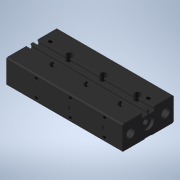
# Autodesk Inventor part: 170831 DFM-12-100-P-A-GF---(Z)
Saved by Autodesk Inventor 2021 (Build 250183000, 183)
## iProperties
Created: 2025-06-15
Part Number: 170831 DFM-12-100-P-A-GF---(Z)
Material: Generic
Catalog Web Link: www.cadenas.de
Description: DFM-(Z)-Guide unit
Vendor: FESTO
Document SubType Name: Modeling
Designer: psAdmin
Manufacturer: FESTO
Mass: 180.298 g
Surface Area: 463.67 cm^2
Volume: 180.298 cm^3
Density: 1 g/cm^3
Appearance: PSOLRGB-175-175-175
Category: PARTsolutions
Company: FESTO
Title: 170831 DFM-12-100-P-A-GF---(Z)
Author: Cadenas PARTsolutions
Comments: Guide unit
PSOL_IDENT_0: {$CADENAS_DATA/23d-libs/festo_fdt/parts/d/dfm/parts/dfm_z.prj},201 {VTYP=3D},{NB=170831 DFM-12-100-P
PSOL_IDENT_1: -A-GF---(Z)},{LINA=170831 DFM-12-100-P-A-GF---(Z)},{NN=DFM-(Z)},{DATE=04.04.2025 09:42:25},{GEOMDATE=
PSOL_IDENT_2: 20.01.2025 12:21:39},{VERSION=},{LINEID=80},{WBVAR=},{WBNUMERIC=}  {NB=170831 DFM-12-100-P-A-GF---(Z
PSOL_IDENT_3: )},{LINA=170831 DFM-12-100-P-A-GF---(Z)},{KT=1},{TNR=170831},{TYP=DFM},{KDM=12},{HUB=100},{F=GF},{BW
PSOL_IDENT_4: E=-},{B1=60.000},{B2=58.000},{B3=42.400},{B4=30.000},{B5=4.500},{B6=51.000},{B7=20.500},{B8=19.000},
PSOL_IDENT_5: {B9=20.000},{B10=20.000},{B11=9.500},{B12=41.000},{B13=19.500},{B14=21.000},{D1=M 5},{D1P=5.000},{D1
PSOL_IDENT_6: KDR=4.134},{D2=8.000},{D3=9.000},{D4=M 4},{D4P=4.000},{D4KDR=3.242},{D5=0.000},{D6=M 4},{D6P=4.000},
PSOL_IDENT_7: {D6KDR=3.242},{D7=10},{D7GF=10.000},{D7KF=8.000},{D8=5.000},{D9=4.300},{FN=1},{FT=GF},{BWET=},{EE=M
PSOL_IDENT_8: 5},{EEMM=5.000},{EEKDR=4.134},{H1=28.050},{H2=26.000},{H3=24.000},{H4=14.050},{H5=14.050},{H6=4.000}
PSOL_IDENT_9: ,{H7=20.000},{H8=0.000},{H9=4.000},{H10=20.000},{H11=14.000},{L1=155.000},{L2=136.000},{L3=10.000},{
PSOL_IDENT_10: L4=13.000},{L5=11.400},{L6=9.500},{L7=6.000},{L8=21.000},{L9=40.000},{L10=34.000},{L11=80.000},{L12=
PSOL_IDENT_11: 11.400},{T1=9.000},{T2=9.400},{T3=2.100},{T4=8.000},{T5=0.000},{T6=1.000},{SW1=14.000},{SW2=11.000},
PSOL_IDENT_12: {SW2D=6.000},{SW2T=3.200},{ZZ=0},{MOD=1},{NA=8.000},{BM=0.000},{BS=0.000},{FE=1.000},{A1=5.000},{A2=
PSOL_IDENT_13: 8.600},{W=30.000},{BR=8.000},{D10=14},{A3=3}
NB: 170831 DFM-12-100-P-A-GF---(Z)
NN: DFM-(Z)
NT: Guide unit
NBSYN: $TNR. $TYP.-$KDM.-$HUB.-P-A-$FT.$BWET.---(Z)
LINA: 170831 DFM-12-100-P-A-GF---(Z)
CATALOG: Festo Design Tool 3D
TNR: 170831
TYP: DFM
KDM: 12
HUB: 100
F: GF
BWE: -
B1: 60
B2: 58
B3: 42.4
B4: 30
B5: 4.5
B6: 51
B7: 20.5
B8: 19
B9: 20
B10: 20
B11: 9.5
B12: 41
B13: 19.5
B14: 21
D1: M 5
D1P: 5
D1KDR: 4.134
D2: 8
D3: 9
D4: M 4
D4P: 4
D4KDR: 3.242
D5: 0
D6: M 4
D6P: 4
D6KDR: 3.242
D7GF: 10
D7KF: 8
D8: 5
D9: 4.3
EE: M 5
EEKDR: 4.134
H1: 28.05
H2: 26
H3: 24
H4: 14.05
H5: 14.05
H6: 4
H7: 20
H8: 0
H9: 4
H10: 20
H11: 14
L1: 155
L2: 136
L3: 10
L4: 13
L5: 11.4
L6: 9.5
L7: 6
L8: 21
L9: 40
L10: 34
L11: 80
L12: 11.4
T1: 9
T2: 9.4
T3: 2.1
T4: 8
T5: 0
T6: 1
SW1: 14
SW2: 11
SW2D: 6
SW2T: 3.2
NA: 8
BM: 0
BS: 0
FE: 1
A1: 5
A2: 8.6
W: 30
BR: 8
SUPPLIER: FESTO
ARTICLENO: 170831 DFM-12-100-P-A-GF---(Z)
BOMINFO: 170831 DFM-12-100-P-A-GF---(Z)
CREATOR: CADENAS GmbH
Autodesk Inventor part; units mm, degrees
ref_plane "YZ Plane" through (0, 0, 0) normal (1, 0, 0) x (0, 1, 0)
ref_plane "XZ Plane" through (0, 0, 0) normal (0, 1, 0) x (-1, 0, 0)
ref_plane "XY Plane" through (0, 0, 0) normal (0, 0, 1) x (1, 0, 0)
sketch "Sketch_1" plane through (0, 0, 0) normal (1, 0, 0) x (0, 1, 0)
  line L0 (14, 30) -> (-14.05, 30)
  line L1 (-14.05, 30) -> (-14.05, -30)
  line L2 (-14.05, -30) -> (14, -30)
  line L3 (14, -30) -> (14, 30)
  constraints: 8 end point
extrude "Extrusion1" add sketch "Sketch_1" against normal blind 136
sketch "Sketch_37" plane through (0, 0, 0) normal (1, 0, 0) x (0, 1, 0)
  line L0 (-40, 60) -> (-40, -60)
  line L1 (-40, -60) -> (40, -60)
  line L2 (40, -60) -> (40, 60)
  line L3 (40, 60) -> (-40, 60)
  line L4 (-13.5, 30) -> (-14.05, 29.45)
  line L5 (-14.05, 29.45) -> (-14.05, 4.0402)
  line L6 (-14.05, 4.0402) -> (-13.5, 3.7226)
  line L7 (-13.5, 3.7226) -> (-13.5, -3.7226)
  line L8 (-13.5, -3.7226) -> (-14.05, -4.0402)
  line L9 (-14.05, -4.0402) -> (-14.05, -28.95)
  line L10 (-14.05, -28.95) -> (-13, -30)
  line L11 (-13, -30) -> (13, -30)
  line L12 (13, -30) -> (14, -29)
  line L13 (14, -29) -> (14, -7)
  arc A0 (14, -7) -> (13.6, -6.6) centre (13.6, -7) ccw
  line L14 (13.6, -6.6) -> (12.4, -6.6)
  arc A1 (12.4, -6.6) -> (12.2, -6.8) centre (12.4, -6.8) ccw
  line L15 (12.2, -6.8) -> (12.2, -7.05)
  arc A2 (12, -7.25) -> (12.2, -7.05) centre (12, -7.05) ccw
  line L16 (12, -7.25) -> (9.4, -7.25)
  arc A3 (9, -6.85) -> (9.4, -7.25) centre (9.4, -6.85) ccw
  line L17 (9, -6.85) -> (9, -1.15)
  arc A4 (9.4, -0.75) -> (9, -1.15) centre (9.4, -1.15) ccw
  line L18 (9.4, -0.75) -> (12, -0.75)
  arc A5 (12.2, -0.95) -> (12, -0.75) centre (12, -0.95) ccw
  line L19 (12.2, -0.95) -> (12.2, -1.2)
  arc A6 (12.2, -1.2) -> (12.4, -1.4) centre (12.4, -1.2) ccw
  line L20 (12.4, -1.4) -> (13.6, -1.4)
  arc A7 (13.6, -1.4) -> (14, -1) centre (13.6, -1) ccw
  line L21 (14, -1) -> (14, 1)
  arc A8 (14, 1) -> (13.6, 1.4) centre (13.6, 1) ccw
  line L22 (13.6, 1.4) -> (12.4, 1.4)
  arc A9 (12.4, 1.4) -> (12.2, 1.2) centre (12.4, 1.2) ccw
  line L23 (12.2, 1.2) -> (12.2, 0.95)
  arc A10 (12, 0.75) -> (12.2, 0.95) centre (12, 0.95) ccw
  line L24 (12, 0.75) -> (9.4, 0.75)
  arc A11 (9, 1.15) -> (9.4, 0.75) centre (9.4, 1.15) ccw
  line L25 (9, 1.15) -> (9, 6.85)
  arc A12 (9.4, 7.25) -> (9, 6.85) centre (9.4, 6.85) ccw
  line L26 (9.4, 7.25) -> (12, 7.25)
  arc A13 (12.2, 7.05) -> (12, 7.25) centre (12, 7.05) ccw
  line L27 (12.2, 7.05) -> (12.2, 6.8)
  arc A14 (12.2, 6.8) -> (12.4, 6.6) centre (12.4, 6.8) ccw
  line L28 (12.4, 6.6) -> (13.6, 6.6)
  arc A15 (13.6, 6.6) -> (14, 7) centre (13.6, 7) ccw
  line L29 (14, 7) -> (14, 29)
  line L30 (14, 29) -> (13, 30)
  line L31 (13, 30) -> (-13.5, 30)
  constraints: 64 end point, 32 point on circle, 16 centre point
extrude "Extrusion2" cut sketch "Sketch_37" against normal blind 136
sketch "Sketch3" plane through (0, 0, 0) normal (1, 0, 0) x (0, 0, -1)
  point P0 (20.5, 0)
hole "Hole1" at (0, 0, -20.5) direction (-1, 0, 0) diameter 10 depth 136
sketch "Sketch4" plane through (0, 0, 0) normal (1, 0, 0) x (0, 0, -1)
  point P0 (-20.5, 0)
hole "Hole2" at (0, 0, 20.5) direction (-1, 0, 0) diameter 10 depth 136
sketch "Sketch5" plane through (-136, 14, -29) normal (0, 1, 0) x (1, 0, 0)
  point P0 (124.6, -16.6)
hole "Hole3" at (-11.4, 14, -12.4) direction (0, -1, 0) diameter 4.134 depth 5 countersink diameter 5 countersink angle 90 thread size "M5x0.8" class "6H" standard "ISO Metric profile"
sketch "Sketch6" plane through (-136, 14, -29) normal (0, 1, 0) x (1, 0, 0)
  point P0 (9.5, -16.6)
hole "Hole4" at (-126.5, 14, -12.4) direction (0, -1, 0) diameter 4.134 depth 5 countersink diameter 5 countersink angle 90 thread size "M5x0.8" class "6H" standard "ISO Metric profile"
sketch "Sketch7" plane through (0, -13, -30) normal (0, 0, -1) x (-1, 0, 0)
  point P0 (11.4, 22.95)
hole "Hole5" at (-11.4, 9.95, -30) direction (0, 0, 1) diameter 4.134 depth 5 countersink diameter 5 countersink angle 90 thread size "M5x0.8" class "6H" standard "ISO Metric profile"
sketch "Sketch8" plane through (0, -13, -30) normal (0, 0, -1) x (-1, 0, 0)
  point P0 (126.5, 22.95)
hole "Hole6" at (-126.5, 9.95, -30) direction (0, 0, 1) diameter 4.134 depth 5 countersink diameter 5 countersink angle 90 thread size "M5x0.8" class "6H" standard "ISO Metric profile"
sketch "Sketch_18" plane through (-21, 0, 0) normal (1, 0, 0) x (0, 0, -1)
  line L0 (9.5, -14.05) -> (9.5, 14)
  line L1 (9.5, 14) -> (13.5, 14)
  line L2 (13.5, 14) -> (13.5, 4.6)
  line L3 (13.5, 4.6) -> (11.65, 4.6)
  line L4 (11.65, 4.6) -> (11.65, -5.05)
  line L5 (11.65, -5.05) -> (10.5, -5.05)
  line L6 (10.5, -5.05) -> (10.5, -11.95)
  line L7 (10.5, -11.95) -> (14, -11.95)
  line L8 (14, -11.95) -> (14, -14.05)
  line L9 (14, -14.05) -> (9.5, -14.05)
  line L10 (9.5, -14.05) -> (9.5, 14)
  constraints: 22 end point
revolve "Revolution1" cut sketch "Sketch_18" angle 360 about axis through (-21, -14.05, -9.5) along (0, 1, 0)
sketch "Sketch_5" plane through (-21, 0, 0) normal (1, 0, 0) x (0, 0, -1)
  line L0 (9.5, -11.95) -> (9.5, -5.05)
  line L1 (9.5, -5.05) -> (11.567, -5.05)
  line L2 (11.567, -5.05) -> (11.567, -11.517)
  line L3 (11.567, -11.517) -> (12, -11.95)
  line L4 (12, -11.95) -> (9.5, -11.95)
  line L5 (9.5, -11.95) -> (9.5, -5.05)
  constraints: 12 end point
revolve "Revolution2" cut sketch "Sketch_5" angle 360 about axis through (-21, -11.95, -9.5) along (0, 1, 0)
thread "Thread1" size "M5x0.8" class "6H" standard "ISO Metric profile" full length
sketch "Sketch_19" plane through (-21, 0, 0) normal (1, 0, 0) x (0, 0, -1)
  line L0 (-9.5, -14.05) -> (-9.5, 14)
  line L1 (-9.5, 14) -> (-5.5, 14)
  line L2 (-5.5, 14) -> (-5.5, 4.6)
  line L3 (-5.5, 4.6) -> (-7.35, 4.6)
  line L4 (-7.35, 4.6) -> (-7.35, -5.05)
  line L5 (-7.35, -5.05) -> (-8.5, -5.05)
  line L6 (-8.5, -5.05) -> (-8.5, -11.95)
  line L7 (-8.5, -11.95) -> (-5, -11.95)
  line L8 (-5, -11.95) -> (-5, -14.05)
  line L9 (-5, -14.05) -> (-9.5, -14.05)
  line L10 (-9.5, -14.05) -> (-9.5, 14)
  constraints: 22 end point
revolve "Revolution3" cut sketch "Sketch_19" angle 360 about axis through (-21, -14.05, 9.5) along (0, 1, 0)
sketch "Sketch_6" plane through (-21, 0, 0) normal (1, 0, 0) x (0, 0, -1)
  line L0 (-9.5, -11.95) -> (-9.5, -5.05)
  line L1 (-9.5, -5.05) -> (-7.433, -5.05)
  line L2 (-7.433, -5.05) -> (-7.433, -11.517)
  line L3 (-7.433, -11.517) -> (-7, -11.95)
  line L4 (-7, -11.95) -> (-9.5, -11.95)
  line L5 (-9.5, -11.95) -> (-9.5, -5.05)
  constraints: 12 end point
revolve "Revolution4" cut sketch "Sketch_6" angle 360 about axis through (-21, -11.95, 9.5) along (0, 1, 0)
thread "Thread2" size "M5x0.8" class "6H" standard "ISO Metric profile" full length
sketch "Sketch_20" plane through (-61, 0, 0) normal (1, 0, 0) x (0, 0, -1)
  line L0 (9.5, -14.05) -> (9.5, 14)
  line L1 (9.5, 14) -> (13.5, 14)
  line L2 (13.5, 14) -> (13.5, 4.6)
  line L3 (13.5, 4.6) -> (11.65, 4.6)
  line L4 (11.65, 4.6) -> (11.65, -5.05)
  line L5 (11.65, -5.05) -> (10.5, -5.05)
  line L6 (10.5, -5.05) -> (10.5, -14.05)
  line L7 (10.5, -14.05) -> (9.5, -14.05)
  line L8 (9.5, -14.05) -> (9.5, 14)
  constraints: 18 end point
revolve "Revolution5" cut sketch "Sketch_20" angle 360 about axis through (-61, -14.05, -9.5) along (0, 1, 0)
sketch "Sketch_7" plane through (-61, 0, 0) normal (1, 0, 0) x (0, 0, -1)
  line L0 (9.5, -14.05) -> (9.5, -5.05)
  line L1 (9.5, -5.05) -> (11.567, -5.05)
  line L2 (11.567, -5.05) -> (11.567, -13.617)
  line L3 (11.567, -13.617) -> (12, -14.05)
  line L4 (12, -14.05) -> (9.5, -14.05)
  line L5 (9.5, -14.05) -> (9.5, -5.05)
  constraints: 12 end point
revolve "Revolution6" cut sketch "Sketch_7" angle 360 about axis through (-61, -14.05, -9.5) along (0, 1, 0)
thread "Thread3" size "M5x0.8" class "6H" standard "ISO Metric profile" full length
sketch "Sketch_21" plane through (-61, 0, 0) normal (1, 0, 0) x (0, 0, -1)
  line L0 (-9.5, -14.05) -> (-9.5, 14)
  line L1 (-9.5, 14) -> (-5.5, 14)
  line L2 (-5.5, 14) -> (-5.5, 4.6)
  line L3 (-5.5, 4.6) -> (-7.35, 4.6)
  line L4 (-7.35, 4.6) -> (-7.35, -5.05)
  line L5 (-7.35, -5.05) -> (-8.5, -5.05)
  line L6 (-8.5, -5.05) -> (-8.5, -14.05)
  line L7 (-8.5, -14.05) -> (-9.5, -14.05)
  line L8 (-9.5, -14.05) -> (-9.5, 14)
  constraints: 18 end point
revolve "Revolution7" cut sketch "Sketch_21" angle 360 about axis through (-61, -14.05, 9.5) along (0, 1, 0)
sketch "Sketch_8" plane through (-61, 0, 0) normal (1, 0, 0) x (0, 0, -1)
  line L0 (-9.5, -14.05) -> (-9.5, -5.05)
  line L1 (-9.5, -5.05) -> (-7.433, -5.05)
  line L2 (-7.433, -5.05) -> (-7.433, -13.617)
  line L3 (-7.433, -13.617) -> (-7, -14.05)
  line L4 (-7, -14.05) -> (-9.5, -14.05)
  line L5 (-9.5, -14.05) -> (-9.5, -5.05)
  constraints: 12 end point
revolve "Revolution8" cut sketch "Sketch_8" angle 360 about axis through (-61, -14.05, 9.5) along (0, 1, 0)
thread "Thread4" size "M5x0.8" class "6H" standard "ISO Metric profile" full length
sketch "Sketch_22" plane through (-101, 0, 0) normal (1, 0, 0) x (0, 0, -1)
  line L0 (9.5, -14.05) -> (9.5, 14)
  line L1 (9.5, 14) -> (13.5, 14)
  line L2 (13.5, 14) -> (13.5, 4.6)
  line L3 (13.5, 4.6) -> (11.65, 4.6)
  line L4 (11.65, 4.6) -> (11.65, -5.05)
  line L5 (11.65, -5.05) -> (10.5, -5.05)
  line L6 (10.5, -5.05) -> (10.5, -14.05)
  line L7 (10.5, -14.05) -> (9.5, -14.05)
  line L8 (9.5, -14.05) -> (9.5, 14)
  constraints: 18 end point
revolve "Revolution9" cut sketch "Sketch_22" angle 360 about axis through (-101, -14.05, -9.5) along (0, 1, 0)
sketch "Sketch_9" plane through (-101, 0, 0) normal (1, 0, 0) x (0, 0, -1)
  line L0 (9.5, -14.05) -> (9.5, -5.05)
  line L1 (9.5, -5.05) -> (11.567, -5.05)
  line L2 (11.567, -5.05) -> (11.567, -13.617)
  line L3 (11.567, -13.617) -> (12, -14.05)
  line L4 (12, -14.05) -> (9.5, -14.05)
  line L5 (9.5, -14.05) -> (9.5, -5.05)
  constraints: 12 end point
revolve "Revolution10" cut sketch "Sketch_9" angle 360 about axis through (-101, -14.05, -9.5) along (0, 1, 0)
thread "Thread5" size "M5x0.8" class "6H" standard "ISO Metric profile" full length
sketch "Sketch_23" plane through (-101, 0, 0) normal (1, 0, 0) x (0, 0, -1)
  line L0 (-9.5, -14.05) -> (-9.5, 14)
  line L1 (-9.5, 14) -> (-5.5, 14)
  line L2 (-5.5, 14) -> (-5.5, 4.6)
  line L3 (-5.5, 4.6) -> (-7.35, 4.6)
  line L4 (-7.35, 4.6) -> (-7.35, -5.05)
  line L5 (-7.35, -5.05) -> (-8.5, -5.05)
  line L6 (-8.5, -5.05) -> (-8.5, -14.05)
  line L7 (-8.5, -14.05) -> (-9.5, -14.05)
  line L8 (-9.5, -14.05) -> (-9.5, 14)
  constraints: 18 end point
revolve "Revolution11" cut sketch "Sketch_23" angle 360 about axis through (-101, -14.05, 9.5) along (0, 1, 0)
sketch "Sketch_10" plane through (-101, 0, 0) normal (1, 0, 0) x (0, 0, -1)
  line L0 (-9.5, -14.05) -> (-9.5, -5.05)
  line L1 (-9.5, -5.05) -> (-7.433, -5.05)
  line L2 (-7.433, -5.05) -> (-7.433, -13.617)
  line L3 (-7.433, -13.617) -> (-7, -14.05)
  line L4 (-7, -14.05) -> (-9.5, -14.05)
  line L5 (-9.5, -14.05) -> (-9.5, -5.05)
  constraints: 12 end point
revolve "Revolution12" cut sketch "Sketch_10" angle 360 about axis through (-101, -14.05, 9.5) along (0, 1, 0)
thread "Thread6" size "M5x0.8" class "6H" standard "ISO Metric profile" full length
sketch "Sketch21" plane through (-136, -13.5, 30) normal (0, 0, 1) x (1, 0, 0)
  point P0 (115, 3.45)
hole "Hole7" at (-21, -10.05, 30) direction (0, 0, -1) diameter 3.242 depth 9.7308 tip angle 120 countersink diameter 4 countersink angle 90 thread size "M4x0.7" class "6H" standard "ISO Metric profile"
sketch "Sketch22" plane through (-136, -13.5, 30) normal (0, 0, 1) x (1, 0, 0)
  point P0 (115, 23.45)
hole "Hole8" at (-21, 9.95, 30) direction (0, 0, -1) diameter 3.242 depth 9.7308 tip angle 120 countersink diameter 4 countersink angle 90 thread size "M4x0.7" class "6H" standard "ISO Metric profile"
sketch "Sketch23" plane through (-136, -13.5, 30) normal (0, 0, 1) x (1, 0, 0)
  point P0 (75, 3.45)
hole "Hole9" at (-61, -10.05, 30) direction (0, 0, -1) diameter 3.242 depth 9.7308 tip angle 120 countersink diameter 4 countersink angle 90 thread size "M4x0.7" class "6H" standard "ISO Metric profile"
sketch "Sketch24" plane through (-136, -13.5, 30) normal (0, 0, 1) x (1, 0, 0)
  point P0 (75, 23.45)
hole "Hole10" at (-61, 9.95, 30) direction (0, 0, -1) diameter 3.242 depth 9.7308 tip angle 120 countersink diameter 4 countersink angle 90 thread size "M4x0.7" class "6H" standard "ISO Metric profile"
sketch "Sketch25" plane through (-136, -13.5, 30) normal (0, 0, 1) x (1, 0, 0)
  point P0 (35, 3.45)
hole "Hole11" at (-101, -10.05, 30) direction (0, 0, -1) diameter 3.242 depth 9.7308 tip angle 120 countersink diameter 4 countersink angle 90 thread size "M4x0.7" class "6H" standard "ISO Metric profile"
sketch "Sketch26" plane through (-136, -13.5, 30) normal (0, 0, 1) x (1, 0, 0)
  point P0 (35, 23.45)
hole "Hole12" at (-101, 9.95, 30) direction (0, 0, -1) diameter 3.242 depth 9.7308 tip angle 120 countersink diameter 4 countersink angle 90 thread size "M4x0.7" class "6H" standard "ISO Metric profile"
sketch "Sketch27" plane through (-136, 0, 0) normal (-1, 0, 0) x (0, 0, 1)
  point P0 (25.5, -10.05)
hole "Hole13" at (-136, -10.05, 25.5) direction (1, 0, 0) diameter 3.242 depth 9.7308 tip angle 120 countersink diameter 4 countersink angle 90 thread size "M4x0.7" class "6H" standard "ISO Metric profile"
sketch "Sketch28" plane through (-136, 0, 0) normal (-1, 0, 0) x (0, 0, 1)
  point P0 (25.5, 9.95)
hole "Hole14" at (-136, 9.95, 25.5) direction (1, 0, 0) diameter 3.242 depth 9.7308 tip angle 120 countersink diameter 4 countersink angle 90 thread size "M4x0.7" class "6H" standard "ISO Metric profile"
sketch "Sketch29" plane through (-136, 0, 0) normal (-1, 0, 0) x (0, 0, 1)
  point P0 (-25.5, -10.05)
hole "Hole15" at (-136, -10.05, -25.5) direction (1, 0, 0) diameter 3.242 depth 9.7308 tip angle 120 countersink diameter 4 countersink angle 90 thread size "M4x0.7" class "6H" standard "ISO Metric profile"
sketch "Sketch30" plane through (-136, 0, 0) normal (-1, 0, 0) x (0, 0, 1)
  point P0 (10.5, -0.05)
hole "Hole16" at (-136, -0.05, 10.5) direction (1, 0, 0) diameter 5 depth 1
sketch "Sketch31" plane through (-136, 0, 0) normal (-1, 0, 0) x (0, 0, 1)
  point P0 (-10.5, -0.05)
hole "Hole17" at (-136, -0.05, -10.5) direction (1, 0, 0) diameter 5 depth 1
sketch "Skizze_1" plane through (0, 0, 0) normal (0, 0, 1) x (1, 0, 0)
  line L0 (0, 0) -> (-117.4, 0)
  line L1 (-117.4, 0) -> (-117.4, 6)
  line L2 (-117.4, 6) -> (-11.4, 6)
  line L3 (-11.4, 6) -> (-11.4, 3)
  line L4 (-11.4, 3) -> (-3, 3)
  line L5 (-3, 3) -> (-3, 7)
  line L6 (-3, 7) -> (0, 7)
  line L7 (0, 7) -> (0, 0)
  line L8 (0, 0) -> (-117.4, 0)
  constraints: 18 end point
revolve "Revolution13" cut sketch "Skizze_1" angle 360 about axis through (0, 0, 0) along (1, 0, 0)
sketch "Skizze_5" plane through (-21, 0, 0) normal (1, 0, 0) x (0, 0, -1)
  line L0 (-29, -0.05) -> (-30, -0.05)
  line L1 (-30, -0.05) -> (-30, 2.45)
  line L2 (-30, 2.45) -> (-29, 2.45)
  line L3 (-29, 2.45) -> (-29, -0.05)
  line L4 (-29, -0.05) -> (-30, -0.05)
  constraints: 10 end point
revolve "Revolution14" cut sketch "Skizze_5" angle 360 about axis through (-21, -0.05, 29) along (0, 0, -1)
sketch "Skizze_6" plane through (-61, 0, 0) normal (1, 0, 0) x (0, 0, -1)
  line L0 (-29, -0.05) -> (-30, -0.05)
  line L1 (-30, -0.05) -> (-30, 2.45)
  line L2 (-30, 2.45) -> (-29, 2.45)
  line L3 (-29, 2.45) -> (-29, -0.05)
  line L4 (-29, -0.05) -> (-30, -0.05)
  constraints: 10 end point
revolve "Revolution15" cut sketch "Skizze_6" angle 360 about axis through (-61, -0.05, 29) along (0, 0, -1)
ref_plane "BP_1_XY" through (-11.4, 14, -12.4) normal (0, 1, 0) x (1, 0, 0)
ref_plane "BP_1_YZ" through (-11.4, 14, -12.4) normal (1, 0, 0) x (0, 0, -1)
ref_plane "BP_1_ZX" through (-11.4, 14, -12.4) normal (0, 0, -1) x (0, 1, 0)
ref_plane "BP_2_XY" through (-126.5, 14, -12.4) normal (0, 1, 0) x (1, 0, 0)
ref_plane "BP_2_YZ" through (-126.5, 14, -12.4) normal (1, 0, 0) x (0, 0, -1)
ref_plane "BP_2_ZX" through (-126.5, 14, -12.4) normal (0, 0, -1) x (0, 1, 0)
ref_plane "DIM_EE_1_TOP_XY" through (-11.4, 14, -12.4) normal (0, -1, 0) x (1, 0, 0)
ref_plane "DIM_EE_1_TOP_YZ" through (-11.4, 14, -12.4) normal (1, 0, 0) x (0, 0, 1)
ref_plane "DIM_EE_1_TOP_ZX" through (-11.4, 14, -12.4) normal (0, 0, 1) x (0, -1, 0)
ref_plane "FDT_ABP1_XY" through (0, 9.75, -4) normal (-1, 0, 0) x (0, 0, -1)
ref_plane "FDT_ABP1_YZ" through (0, 9.75, -4) normal (0, 0, -1) x (0, -1, 0)
ref_plane "FDT_ABP1_ZX" through (0, 9.75, -4) normal (0, -1, 0) x (-1, 0, 0)
ref_plane "FDT_ABP2_XY" through (0, 9.75, 4) normal (-1, 0, 0) x (0, 0, -1)
ref_plane "FDT_ABP2_YZ" through (0, 9.75, 4) normal (0, 0, -1) x (0, -1, 0)
ref_plane "FDT_ABP2_ZX" through (0, 9.75, 4) normal (0, -1, 0) x (-1, 0, 0)
ref_plane "FDT_QSFRONT_XY" through (-11.4, 14, -12.4) normal (0, 1, 0) x (0, 0, -1)
ref_plane "FDT_QSFRONT_YZ" through (-11.4, 14, -12.4) normal (0, 0, -1) x (-1, 0, 0)
ref_plane "FDT_QSFRONT_ZX" through (-11.4, 14, -12.4) normal (-1, 0, 0) x (0, 1, 0)
ref_plane "FDT_QSREAR_XY" through (-126.5, 14, -12.4) normal (0, 1, 0) x (0, 0, -1)
ref_plane "FDT_QSREAR_YZ" through (-126.5, 14, -12.4) normal (0, 0, -1) x (-1, 0, 0)
ref_plane "FDT_QSREAR_ZX" through (-126.5, 14, -12.4) normal (-1, 0, 0) x (0, 1, 0)
ref_plane "FDT_QS_SIDE_FRONT_XY" through (-11.4, 9.95, -30) normal (0, 0, -1) x (0, -1, 0)
ref_plane "FDT_QS_SIDE_FRONT_YZ" through (-11.4, 9.95, -30) normal (0, -1, 0) x (-1, 0, 0)
ref_plane "FDT_QS_SIDE_FRONT_ZX" through (-11.4, 9.95, -30) normal (-1, 0, 0) x (0, 0, -1)
ref_plane "FDT_QS_SIDE_REAR_XY" through (-126.5, 9.95, -30) normal (0, 0, -1) x (0, -1, 0)
ref_plane "FDT_QS_SIDE_REAR_YZ" through (-126.5, 9.95, -30) normal (0, -1, 0) x (-1, 0, 0)
ref_plane "FDT_QS_SIDE_REAR_ZX" through (-126.5, 9.95, -30) normal (-1, 0, 0) x (0, 0, -1)
ref_plane "FDT_SLOT1_XY" through (-68, 9, -4) normal (0, 1, 0) x (0, 0, -1)
ref_plane "FDT_SLOT1_YZ" through (-68, 9, -4) normal (0, 0, -1) x (-1, 0, 0)
ref_plane "FDT_SLOT1_ZX" through (-68, 9, -4) normal (-1, 0, 0) x (0, 1, 0)
ref_plane "FDT_SLOT2_XY" through (-68, 9, 4) normal (0, 1, 0) x (0, 0, -1)
ref_plane "FDT_SLOT2_YZ" through (-68, 9, 4) normal (0, 0, -1) x (-1, 0, 0)
ref_plane "FDT_SLOT2_ZX" through (-68, 9, 4) normal (-1, 0, 0) x (0, 1, 0)
ref_plane "HUELSE1_1_XY" through (-135, -0.05, 10.5) normal (1, 0, 0) x (0, 0, -1)
ref_plane "HUELSE1_1_YZ" through (-135, -0.05, 10.5) normal (0, 0, -1) x (0, 1, 0)
ref_plane "HUELSE1_1_ZX" through (-135, -0.05, 10.5) normal (0, 1, 0) x (1, 0, 0)
ref_plane "HUELSE1_2_XY" through (-135, -0.05, -10.5) normal (1, 0, 0) x (0, 0, -1)
ref_plane "HUELSE1_2_YZ" through (-135, -0.05, -10.5) normal (0, 0, -1) x (0, 1, 0)
ref_plane "HUELSE1_2_ZX" through (-135, -0.05, -10.5) normal (0, 1, 0) x (1, 0, 0)
ref_plane "HUELSE2_1_XY" through (-21, -11.95, -9.5) normal (0, 1, 0) x (1, 0, 0)
ref_plane "HUELSE2_1_YZ" through (-21, -11.95, -9.5) normal (1, 0, 0) x (0, 0, -1)
ref_plane "HUELSE2_1_ZX" through (-21, -11.95, -9.5) normal (0, 0, -1) x (0, 1, 0)
ref_plane "HUELSE2_2_XY" through (-21, -11.95, 9.5) normal (0, 1, 0) x (1, 0, 0)
ref_plane "HUELSE2_2_YZ" through (-21, -11.95, 9.5) normal (1, 0, 0) x (0, 0, -1)
ref_plane "HUELSE2_2_ZX" through (-21, -11.95, 9.5) normal (0, 0, -1) x (0, 1, 0)
ref_plane "TO_DUMMY_XY" through (0, 0, 0) normal (0, 1, 0) x (0, 0, 1)
ref_plane "TO_DUMMY_YZ" through (0, 0, 0) normal (0, 0, 1) x (1, 0, 0)
ref_plane "TO_DUMMY_ZX" through (0, 0, 0) normal (1, 0, 0) x (0, 1, 0)
ref_plane "dfm_z_XY" through (0, 0, 0) normal (1, 0, 0) x (0, 0, -1)
ref_plane "dfm_z_YZ" through (0, 0, 0) normal (0, 0, -1) x (0, 1, 0)
ref_plane "dfm_z_ZX" through (0, 0, 0) normal (0, 1, 0) x (1, 0, 0)
body "Solid1"
